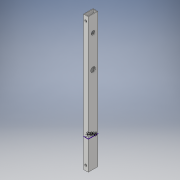
# Autodesk Inventor part: 2x1 16in Aluminum-ver1-1111-2020
Saved by Autodesk Inventor 2018 (Build 220112000, 112)
## iProperties
Created: 2020-01-28
Part Number: 2x1 16in Aluminum-ver1-1111-2020
Material: Generic
Document SubType Name: Modeling
Designer: JMHal
Density: 1 g/cm^3
Appearance: Default
Author: JMHal
Autodesk Inventor part; units mm, degrees
ref_plane "YZ Plane" through (0, 0, 0) normal (1, 0, 0) x (0, 1, 0)
ref_plane "XZ Plane" through (0, 0, 0) normal (0, 1, 0) x (-1, 0, 0)
ref_plane "XY Plane" through (0, 0, 0) normal (0, 0, 1) x (1, 0, 0)
sketch "Sketch1" plane through (0, 0, 0) normal (0, 1, 0) x (-1, 0, 0)
  line L0 (0, 0) -> (25.4, 0)
  line L1 (25.4, 0) -> (25.4, -50.8)
  line L2 (25.4, -50.8) -> (0, -50.8)
  line L3 (0, -50.8) -> (0, 0)
  line L4 (22.225, -47.625) -> (22.225, -3.175)
  line L5 (22.225, -3.175) -> (3.175, -3.175)
  line L6 (3.175, -3.175) -> (3.175, -47.625)
  line L7 (3.175, -47.625) -> (22.225, -47.625)
  dimension "d0" = 50.8
  dimension "d1" = 25.4
  dimension "d2" = 3.175
  constraints: 16 end point, 4 parallel, 2 perpendicular, 1 horizontal, 3 other
  measures "d0" distance between parallel lines of L2 L0
  measures "d1" distance between parallel lines of L1 L3
  measures "d2" distance between parallel lines of L1 L4
extrude "Extrusion1" add sketch "Sketch1" along normal blind 558.8
sketch "Sketch2" plane through (0, 0, 0) normal (1, 0, 0) x (0, 0, -1)
  circle A0 centre (25.4, 304.8) radius 12.7
  line L0 (0, 0) -> (0, 558.8) projected
  line L1 (50.8, 0) -> (0, 0) projected
  line L2 (50.8, 558.8) -> (0, 558.8) projected
  dimension "d5" = 25.4
  dimension "d6" = 25.4
  dimension "d24" = 254
  constraints: 1 centre point
  measures "d5" diameter of A0
  measures "d6" distance from line of A0.centre L0
  measures "d24" distance from line of L2 A0.centre
extrude "Extrusion2" cut sketch "Sketch2" against normal blind 25.4
sketch "Sketch4" plane through (-22.225, 0, -47.625) normal (1, 0, 0) x (0, 0, -1)
  circle A0 centre (-22.225, 473.075) radius 7.62
  line L0 (-47.625, 558.8) -> (3.175, 558.8) projected
  line L1 (-47.625, 0) -> (-47.625, 558.8) projected
  dimension "d15" = 25.4
  dimension "d16" = 15.24
  dimension "d20" = 85.725
  constraints: 1 centre point
  measures "d15" distance from line of L1 A0.centre
  measures "d16" diameter of A0
  measures "d20" distance from line of L0 A0.centre
extrude "Extrusion4" cut sketch "Sketch4" against normal blind 12.7
extrude "Extrusion5" add sketch "Sketch1" against normal blind 152.4
sketch "Sketch8" plane through (-25.4, 558.8, -50.8) normal (-1, 0, 0) x (0, 0, 1)
  line L0 (47.625, -63.5) -> (3.175, -63.5)
  line L1 (3.175, -63.5) -> (3.175, -107.95)
  line L2 (3.175, -107.95) -> (47.625, -107.95)
  line L3 (47.625, -107.95) -> (47.625, -63.5)
  line L4 (0, 0) -> (50.8, 0) projected
  line L5 (47.625, -711.2) -> (47.625, 0) projected
  line L6 (3.175, 0) -> (3.175, -711.2) projected
  point P0 (50.8, -558.8)
  dimension "d29" = 63.5
  dimension "d30" = 0
  dimension "d31" = 0
  dimension "d32" = 44.45
  constraints: 8 end point, 2 parallel, 1 horizontal, 1 perpendicular
  measures "d29" distance between parallel lines of L4 L0
  measures "d30" distance between parallel lines of L5 L3
  measures "d31" distance between parallel lines of L6 L1
  measures "d32" distance between parallel lines of L0 L2
extrude "Extrusion6" cut sketch "Sketch8" against normal blind 12.7 contours L3 L2 L1 L0
sketch "Sketch9" plane through (0, 558.8, 0) normal (1, 0, 0) x (0, 0, -1)
  circle A0 centre (25.4, -85.725) radius 10.16
  line L0 (0, 0) -> (50.8, 0) projected
  line L1 (50.8, 0) -> (50.8, -711.2) projected
  point P0 (0, -558.8)
  dimension "d35" = 85.725
  dimension "d36" = 25.4
  dimension "d37" = 20.32
  constraints: 1 centre point
  measures "d35" distance from line of L0 A0.centre
  measures "d36" distance from line of L1 A0.centre
  measures "d37" diameter of A0
extrude "Extrusion7" cut sketch "Sketch9" against normal blind 12.7
sketch "Sketch11" plane through (0, 558.8, -50.8) normal (0, 0, -1) x (-1, 0, 0)
  circle A0 centre (12.7, -25.4) radius 5.715
  line L0 (0, 0) -> (25.4, 0) projected
  line L1 (25.4, 0) -> (25.4, -711.2) projected
  circle A1 centre (12.7, -685.8) radius 5.715
  line L2 (25.4, -711.2) -> (0, -711.2) projected
  point P0 (0, -558.8)
  dimension "d48" = 11.43
  dimension "d49" = 25.4
  dimension "d50" = 12.7
  dimension "d51" = 11.43
  dimension "d52" = 12.7
  dimension "d53" = 25.4
  constraints: 2 centre point
  measures "d48" diameter of A0
  measures "d49" distance from line of A0.centre L0
  measures "d50" distance from line of A0.centre L1
  measures "d51" diameter of A1
  measures "d52" distance from line of A1.centre L1
  measures "d53" distance from line of A1.centre L2
extrude "Extrusion9" cut sketch "Sketch11" against normal blind 50.8
body "Solid1"
